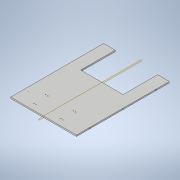
# Autodesk Inventor part: main plate
Saved by Autodesk Inventor 2021 (Build 250183000, 183)
## iProperties
Created: 2020-10-03
Part Number: main plate
Material: Generic
Document SubType Name: Modeling
Designer: User
Density: 1 g/cm^3
Appearance: Default
Author: User
Autodesk Inventor part; units mm, degrees
ref_plane "YZ Plane" through (0, 0, 0) normal (1, 0, 0) x (0, 1, 0)
ref_plane "XZ Plane" through (0, 0, 0) normal (0, 1, 0) x (-1, 0, 0)
ref_plane "XY Plane" through (0, 0, 0) normal (0, 0, 1) x (1, 0, 0)
sketch "Sketch1" plane through (0, 0, 0) normal (0, 1, 0) x (-1, 0, 0)
  line L0 (0, 0) -> (314.96, 0)
  line L1 (314.96, 0) -> (314.96, -444.5)
  line L2 (314.96, -444.5) -> (0, -444.5)
  line L3 (0, -444.5) -> (0, 0)
  dimension "d0" = 314.96
  dimension "d1" = 444.5
  constraints: 8 end point, 2 parallel, 1 horizontal, 1 perpendicular
  measures "d0" distance of L1.end L2.end
  measures "d1" distance of L0.end L1.end
extrude "Extrusion1" add sketch "Sketch1" along normal blind 6.35
sketch "Sketch2" plane through (0, 6.35, 0) normal (0, 1, 0) x (1, 0, 0)
  circle A0 centre (-95.1484, 30.099) radius 1.3589
  circle A1 centre (-105.156, 30.099) radius 1.3589
  line L0 (-314.96, 0) -> (0, 0) projected
  line L1 (0, 0) -> (0, 444.5) projected
  dimension "d4" = 2.7178
  dimension "d5" = 2.7178
  dimension "d7" = 95.1484
  dimension "d8" = 10.0076
  dimension "d9" = 30.099
  dimension "d37" = 30.099
  constraints: 2 centre point
  measures "d4" diameter of A0
  measures "d5" diameter of A1
  measures "d7" distance from line of L1 A0.centre
  measures "d8" distance of A1.centre A0.centre
  measures "d9" distance from line of L0 A1.centre
  measures "d37" distance from line of L0 A0.centre
extrude "Extrusion2" cut sketch "Sketch2" against normal blind 25.4
sketch "Sketch3" plane through (0, 6.35, 0) normal (0, 1, 0) x (1, 0, 0)
  circle A0 centre (-107.696, 93.1418) radius 1.3589
  circle A1 centre (-97.6884, 93.1418) radius 1.3589
  circle A2 centre (-95.1484, 30.099) radius 1.3589 projected
  circle A3 centre (-105.156, 30.099) radius 1.3589 projected
  line L0 (0, 0) -> (0, 444.5) projected
  dimension "d12" = 2.7178
  dimension "d13" = 2.7178
  dimension "d14" = 63.0428
  dimension "d15" = 63.0428
  dimension "d16" = 10.0076
  dimension "d17" = 97.6884
  constraints: 2 centre point
  measures "d12" diameter of A0
  measures "d13" diameter of A1
  measures "d14" vertical distance of A1.centre A2.centre
  measures "d15" vertical distance of A3.centre A0.centre
  measures "d16" distance of A0.centre A1.centre
  measures "d17" distance from line of L0 A1.centre
extrude "Extrusion3" cut sketch "Sketch3" against normal blind 25.4 contours A0 | A1
sketch "Sketch4" plane through (0, 6.35, 0) normal (0, 1, 0) x (1, 0, 0)
  circle A0 centre (-240.5634, 93.091) radius 1.3589
  circle A1 centre (-230.5562, 93.1789) radius 1.3589
  line L0 (-314.96, 444.5) -> (-314.96, 0) projected
  line L1 (-314.96, 0) -> (0, 0) projected
  dimension "d20" = 2.7178
  dimension "d21" = 2.7178
  dimension "d22" = 10.0076
  dimension "d23" = 74.3966
  dimension "d24" = 93.091
  constraints: 2 centre point
  measures "d20" diameter of A0
  measures "d21" diameter of A1
  measures "d22" distance of A1.centre A0.centre
  measures "d23" distance from line of L0 A0.centre
  measures "d24" distance from line of L1 A0.centre
extrude "Extrusion4" cut sketch "Sketch4" against normal blind 25.4
sketch "Sketch5" plane through (0, 6.35, 0) normal (0, 1, 0) x (1, 0, 0)
  circle A0 centre (-232.029, 28.702) radius 1.3589
  circle A1 centre (-222.0214, 28.702) radius 1.3589
  line L0 (-314.96, 0) -> (0, 0) projected
  line L1 (-314.96, 444.5) -> (-314.96, 0) projected
  line L2 (0, 0) -> (0, 444.5) projected
  dimension "d27" = 2.7178
  dimension "d28" = 2.7178
  dimension "d31" = 28.702
  dimension "d32" = 10.0076
  dimension "d36" = 222.0214
  dimension "d38" = 28.702
  constraints: 2 centre point
  measures "d27" diameter of A0
  measures "d28" diameter of A1
  measures "d31" distance from line of L0 A0.centre
  measures "d32" distance of A1.centre A0.centre
  measures "d36" distance from line of L2 A1.centre
  measures "d38" distance from line of L0 A1.centre
extrude "Extrusion5" cut sketch "Sketch5" against normal blind 25.4
sketch "Sketch6" plane through (0, 0, 0) normal (1, 0, 0) x (0, 0, -1)
  line L0 (444.5, 0) -> (444.5, 6.35) projected
  line L1 (0, 6.35) -> (444.5, 6.35) projected
  line L2 (0, 0) -> (0, 6.35) projected
  point P0 (63.5, 3.175)
  point P1 (222.25, 3.175)
  point P2 (381, 3.175)
  dimension "d39" = 6.35
  dimension "d40" = 3.175
  dimension "d41" = 3.175
  dimension "d42" = 3.175
  dimension "d43" = 63.5
  dimension "d44" = 63.5
  dimension "d45" = 317.5
  dimension "d46" = 158.75
  measures "d39" distance of L0.start L0.end
  measures "d40" distance from line of L1 point (381, 3.175)
  measures "d41" distance from line of L1 point (222.25, 3.175)
  measures "d42" distance from line of L1 point (63.5, 3.175)
  measures "d43" distance from line of point (63.5, 3.175) L2
  measures "d44" distance from line of L0 point (381, 3.175)
  measures "d45" distance of point (381, 3.175) point (63.5, 3.175)
  measures "d46" distance of point (222.25, 3.175) point (63.5, 3.175)
hole "Hole1" at (0, 3.175, -63.5) at (0, 3.175, -222.25) at (0, 3.175, -381) direction (-1, 0, 0) diameter 4.9784 depth 19.05 tip angle 118 thread size "1/4-20 UNC" class "2B" standard "ANSI Unified Screw Threads"
ref_plane "Work Plane1" through (-157.48, 0, 0) normal (1, 0, 0) x (0, 0, -1)
mirror "Mirror1" about plane through (-157.48, 0, 0) normal (1, 0, 0) of "Hole1"
sketch "Sketch7" plane through (0, 6.35, 0) normal (0, 1, 0) x (1, 0, 0)
  line L0 (0, 444.5) -> (-314.96, 444.5) projected
  line L1 (-55.88, 444.5) -> (-259.08, 444.5)
  line L2 (-259.08, 444.5) -> (-259.08, 279.4)
  line L3 (-259.08, 279.4) -> (-55.88, 279.4)
  line L4 (-55.88, 279.4) -> (-55.88, 444.5)
  line L5 (-314.96, 444.5) -> (-314.96, 0) projected
  point P0 (0, 0)
  dimension "d54" = 203.2
  dimension "d55" = 165.1
  dimension "d56" = 55.88
  constraints: 8 end point, 2 parallel, 1 horizontal, 1 perpendicular, 1 point on line
  measures "d54" distance of L3.end L2.end
  measures "d55" distance of L2.end L1.end
  measures "d56" distance between parallel lines of L5 L2
extrude "Extrusion6" cut sketch "Sketch7" against normal through all
equation "\"d40\" = 0.5 * d39"
equation "\"d41\" = d40"
equation "\"d42\" = d41"
equation "\"d44\" = d43"
equation "\"d46\" = 0.5 * d45"
body "Solid1"
